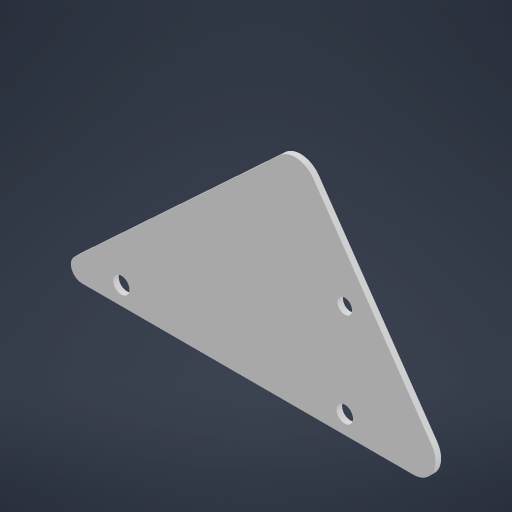
# Autodesk Inventor part: tangentsled
Saved by Autodesk Inventor 2024.2 (Build 282272000, 272)
## iProperties
Created: 2024-01-01
Part Number: tangentsled
Material: Generic
Document SubType Name: Modeling
Designer: reima
Density: 1 g/cm^3
Appearance: Default
Author: reima
Autodesk Inventor part; units mm, degrees
ref_plane "YZ Plane" through (0, 0, 0) normal (1, 0, 0) x (0, 1, 0)
ref_plane "XZ Plane" through (0, 0, 0) normal (0, 1, 0) x (-1, 0, 0)
ref_plane "XY Plane" through (0, 0, 0) normal (0, 0, 1) x (1, 0, 0)
sketch "Sketch1" plane through (0, 0, 0) normal (0, 0, 1) x (1, 0, 0)
  circle A0 centre (425.45, 20.65) radius 2.0828 projected
  circle A1 centre (425.45, 20.65) radius 34.925 construction
  line L0 (425.45, 55.575) -> (298.45, 55.575) construction
  line L1 (323.85, 55.575) -> (323.85, 42.875) construction
  circle A2 centre (323.85, 12.649) radius 30.226 construction
  circle A3 centre (425.45, 20.65) radius 33.02 construction
  line L2 (406.9994, 48.5755) -> (348.6303, -5.5907)
  line L3 (420.1242, 27) -> (481.5758, 27) projected
  line L4 (442.214, -11.1) -> (383.027, -11.1) projected
  line L5 (450.1296, -1.1362) -> (416.5451, 47.5277)
  circle A4 centre (425.45, 20.65) radius 7.9375 construction
  arc A5 (416.5451, 47.5277) -> (406.9994, 48.5755) centre (411.3189, 43.9209) ccw
  line L6 (444.9034, -11.093) -> (350.7901, -11.093)
  line L7 (457.0011, -11.093) -> (551.1145, -11.093) construction
  arc A6 (444.9034, -11.093) -> (450.1296, -1.1362) centre (444.9034, -4.743) ccw
  arc A7 (348.6303, -5.5907) -> (350.7901, -11.093) centre (350.7901, -7.918) ccw
  circle A8 centre (387.35, -5.9184) radius 2.3114 projected
  circle A9 centre (361.95, -5.9184) radius 2.3114 projected
  circle A10 centre (438.15, -5.9184) radius 2.3114 projected
  circle A11 centre (425.45, -5.9184) radius 2.3368
  point P0 (0, 0)
  point P1 (342.7011, -11.093)
  dimension "d0" = 69.85
  dimension "d1" = 127
  dimension "d2" = 12.7
  dimension "d3" = 60.452
  dimension "d4" = 30.226
  dimension "d5" = 101.6
  dimension "d6" = 66.04
  dimension "d9" = 15.875
  dimension "d10" = 6.35
  dimension "d11" = 180
  dimension "d12" = 114.3
  dimension "d13" = 6.35
  dimension "d14" = 3.175
  dimension "d15" = 5.1746
  dimension "d16" = 101.6
  dimension "d19" = 4.6736
  dimension "d20" = 12.7
  constraints: 12 end point, 9 tangent, 7 centre point, 6 point on circle, 5 point on line, 3 coincident, 3 horizontal, 1 collinear, 1 vertical, 1 vertical alignment, 2 other
  measures "d1" distance of L0.start L0.end
  measures "d2" distance of L1.start L1.end
  measures "d3" diameter of A2
  measures "d4" distance of A2.centre L1.end
  measures "d5" distance from line of A0.centre L1
  measures "d6" diameter of A3
  measures "d9" diameter of A4
  measures "d10" radius of A5
  measures "d11" angle of L6 L7
  measures "d12" distance of L7.start point (342.701, -11.093)
  measures "d13" radius of A6
  measures "d14" radius of A7
  measures "d15" distance from line of A8.centre L6
  measures "d16" horizontal distance of A2.centre A0.centre
  measures "d19" diameter of A11
  measures "d20" distance of A11.centre A10.centre
extrude "Extrusion1" add sketch "Sketch1" along normal blind 1.5875 contours A5 L5 A6 L6 A7 L2 | A8 | A10 | A11
extrude "Extrusion2" cut sketch "Sketch1" along normal blind 1.5875 contours A11
body "Solid1"
